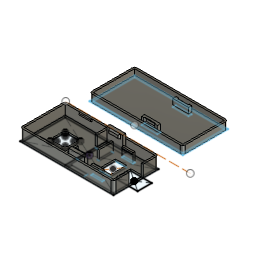
co2_01space_box (Autodesk Fusion 360 design; units mm, degrees)
Autodesk Fusion 360 part; units mm, degrees
sketch "Sketch7" plane through (0, 0, 0) normal (0, 0, 1) x (1, 0, 0)
  line L0 (28.4, 13.1) -> (-28.4, 13.1)
  line L1 (-28.4, 13.1) -> (-28.4, -13.1)
  line L2 (-28.4, -13.1) -> (28.4, -13.1)
  line L3 (28.4, -13.1) -> (28.4, 13.1)
  line L4 (28.4, 13.1) -> (-28.4, -13.1) construction
  line L5 (-28.4, 13.1) -> (28.4, -13.1) construction
  line L6 (-29.6, -14.3) -> (29.6, -14.3)
  line L7 (29.6, -14.3) -> (29.6, 14.3)
  line L8 (29.6, 14.3) -> (-29.6, 14.3)
  line L9 (-29.6, 14.3) -> (-29.6, -14.3)
  line L10 (-28.4, 13.1) -> (-2.2, 13.1)
  line L11 (-2.2, 13.1) -> (-2.2, -13.1)
  line L12 (-2.2, -13.1) -> (-28.4, -13.1)
  line L13 (-28.4, -13.1) -> (-28.4, 13.1)
  line L14 (-18.1, 4.8) -> (-12.5, 4.8)
  line L15 (-10.5, 2.8) -> (-10.5, -2.8)
  line L16 (-12.5, -4.8) -> (-18.1, -4.8)
  line L17 (-20.1, -2.8) -> (-20.1, 2.8)
  arc A0 (-18.1, 4.8) -> (-20.1, 2.8) centre (-18.1, 2.8) ccw
  arc A1 (-10.5, 2.8) -> (-12.5, 4.8) centre (-12.5, 2.8) ccw
  arc A2 (-20.1, -2.8) -> (-18.1, -4.8) centre (-18.1, -2.8) ccw
  arc A3 (-12.5, -4.8) -> (-10.5, -2.8) centre (-12.5, -2.8) ccw
  line L18 (-2.2, 13.1) -> (-1, 13.1)
  line L19 (-1, 13.1) -> (-1, -13.1)
  line L20 (-1, -13.1) -> (-2.2, -13.1)
  line L21 (-2.2, -13.1) -> (-2.2, 13.1)
  line L22 (-2.2, 5.9651) -> (-1, 5.9651)
  line L23 (-1, 5.9651) -> (-1, -6)
  line L24 (-1, -6) -> (-2.2, -6)
  line L25 (-2.2, -6) -> (-2.2, 5.9651)
  line L26 (35.1, -4.5) -> (21.7, -4.5)
  line L27 (21.7, -4.5) -> (21.7, 4.5)
  line L28 (21.7, 4.5) -> (35.1, 4.5)
  line L29 (35.1, 4.5) -> (35.1, -4.5)
  line L30 (35.1, -4.5) -> (21.7, 4.5) construction
  line L31 (21.7, -4.5) -> (35.1, 4.5) construction
  line L32 (18.5, -5) -> (11.5, -5)
  line L33 (11.5, -5) -> (11.5, 5)
  line L34 (11.5, 5) -> (18.5, 5)
  line L35 (18.5, 5) -> (18.5, -5)
  line L36 (18.5, -5) -> (11.5, 5) construction
  line L37 (11.5, -5) -> (18.5, 5) construction
  line L38 (11.5, 10.4) -> (18.5, 10.4)
  line L39 (18.5, 10.4) -> (18.5, 9.2)
  line L40 (18.5, 9.2) -> (11.5, 9.2)
  line L41 (11.5, 9.2) -> (11.5, 10.4)
  line L42 (11.5, -9.2) -> (18.5, -9.2)
  line L43 (18.5, -9.2) -> (18.5, -10.4)
  line L44 (18.5, -10.4) -> (11.5, -10.4)
  line L45 (11.5, -10.4) -> (11.5, -9.2)
  line L46 (6.2, 0) -> (5, 0)
  line L47 (5, 0) -> (5, 9)
  line L48 (5, 9) -> (6.2, 9)
  line L49 (6.2, 9) -> (6.2, 0)
  line L50 (-37, 22) -> (42, 22) construction
  line L51 (0, 13.1) -> (10, 13.1)
  line L52 (10, 13.1) -> (10, 11.1)
  line L53 (10, 11.1) -> (0, 11.1)
  line L54 (0, 11.1) -> (0, 13.1)
  line L55 (0, -13.1) -> (10, -13.1)
  line L56 (10, -13.1) -> (10, -11.1)
  line L57 (10, -11.1) -> (0, -11.1)
  line L58 (0, -11.1) -> (0, -13.1)
  line L59 (-29.6, 29.7) -> (-29.6, 58.3)
  line L60 (29.6, 29.7) -> (-29.6, 29.7)
  line L61 (-28.4, 30.9) -> (-2.2, 30.9)
  line L62 (-28.4, 30.9) -> (-28.4, 57.1)
  line L63 (-28.4, 57.1) -> (28.4, 57.1)
  line L64 (-29.6, 58.3) -> (29.6, 58.3)
  line L65 (29.6, 58.3) -> (29.6, 29.7)
  line L66 (28.4, 57.1) -> (28.4, 30.9)
  line L67 (28.4, 30.9) -> (-28.4, 30.9)
  line L68 (0, 33.1) -> (10, 33.1)
  line L69 (10, 33.1) -> (10, 35.1)
  line L70 (10, 35.1) -> (0, 35.1)
  line L71 (0, 35.1) -> (0, 33.1)
  line L72 (0, 54.9) -> (10, 54.9)
  line L73 (10, 54.9) -> (10, 52.9)
  line L74 (10, 52.9) -> (0, 52.9)
  line L75 (0, 52.9) -> (0, 54.9)
  point P0 (-20.1, 4.8)
  point P1 (-10.5, 4.8)
  point P2 (-20.1, -4.8)
  point P3 (28.4, 0)
  point P4 (15, 0)
  dimension "d75" = 56.8
  dimension "d76" = 26.2
  dimension "d77" = 1.2
  dimension "d78" = 26.2
  dimension "d79" = 26.2
  dimension "d80" = 9.6
  dimension "d81" = 9.6
  dimension "d82" = 8.3
  dimension "d83" = 8.3
  dimension "d84" = 2
  dimension "d85" = 2
  dimension "d86" = 2
  dimension "d87" = 2
  dimension "d88" = 1.2
  dimension "d89" = 26.2
  dimension "d90" = 1.2
  dimension "d91" = 11.9651
  dimension "d92" = 13.4
  dimension "d93" = 9
  dimension "d94" = 7
  dimension "d95" = 10
  dimension "d96" = 6.7
  dimension "d101" = 7
  dimension "d102" = 1.2
  dimension "d103" = 4.2
  dimension "d104" = 7
  dimension "d105" = 1.2
  dimension "d106" = 4.2
  dimension "d107" = 1.2
  dimension "d108" = 9
  dimension "d109" = 5.3
  dimension "d131" = 10
  dimension "d132" = 2
  dimension "d133" = 2
  dimension "d134" = 2
  dimension "d135" = 10
  dimension "d136" = 2
  dimension "d143" = 2.2
  dimension "d144" = 2.2
  constraint horizontal L0
  constraint perpendicular L0 L1
  constraint parallel L0 L2
  constraint parallel L1 L3
  constraint coincident L4 origin
  constraint coincident L5 origin
  constraint horizontal L10
  constraint vertical L11
  constraint horizontal L12
  constraint vertical L13
  constraint horizontal L14
  constraint vertical L15
  constraint horizontal L16
  constraint vertical L17
  constraint coincident P0 L17
  constraint coincident P0 L14
  constraint tangent L17 A0
  constraint tangent L14 A0
  constraint coincident P1 L14
  constraint coincident P1 L15
  constraint tangent L14 A1
  constraint tangent L15 A1
  constraint coincident P2 L17
  constraint coincident P2 L16
  constraint tangent L17 A2
  constraint tangent L16 A2
  constraint tangent L16 A3
  constraint tangent L15 A3
  constraint horizontal L18
  constraint vertical L19
  constraint horizontal L20
  constraint vertical L21
  constraint horizontal L22
  constraint vertical L23
  constraint horizontal L24
  constraint vertical L25
  constraint coincident L11 L22.start
  constraint horizontal L26
  constraint perpendicular L26 L27
  constraint parallel L26 L28
  constraint parallel L27 L29
  constraint coincident L30 P3
  constraint coincident L31 P3
  constraint midpoint L3 P3
  constraint horizontal L32
  constraint perpendicular L32 L33
  constraint parallel L32 L34
  constraint parallel L33 L35
  constraint coincident L36 P4
  constraint coincident L37 P4
  constraint horizontal L38
  constraint vertical L39
  constraint horizontal L40
  constraint vertical L41
  constraint horizontal L42
  constraint vertical L43
  constraint horizontal L44
  constraint vertical L45
  constraint horizontal L46
  constraint vertical L47
  constraint horizontal L48
  constraint vertical L49
  constraint parallel L8 L50
  constraint horizontal L51
  constraint vertical L52
  constraint horizontal L53
  constraint vertical L54
  constraint midpoint L0 L51.start
  constraint horizontal L55
  constraint vertical L56
  constraint horizontal L57
  constraint vertical L58
  constraint midpoint L2 L55.start
  constraint symmetric L0.start L50 L66.end
  constraint symmetric L0.end L50 L61.start
  constraint symmetric L1.end L50 L62.end
  constraint symmetric L2.end L50 L63.end
  constraint symmetric L6.start L50 L59.end
  constraint symmetric L6.end L50 L64.end
  constraint symmetric L7.end L50 L60.start
  constraint symmetric L8.end L50 L59.start
  constraint symmetric L10.end L50 L61.end
  constraint horizontal L68
  constraint vertical L69
  constraint horizontal L70
  constraint vertical L71
  constraint horizontal L72
  constraint vertical L73
  constraint horizontal L74
  constraint vertical L75
  measures "d75" distance of L1.end L2.end
  measures "d76" distance of L0.end L1.end
  measures "d78" distance of L0.end L10.end
  measures "d79" distance of L0.end L1.end
  measures "d80" distance of P0 P1
  measures "d81" distance of P0 P2
  measures "d82" distance of L0 L14
  measures "d83" distance of L13 L17
  measures "d84" radius of A0
  measures "d85" radius of A1
  measures "d86" radius of A2
  measures "d87" radius of A3
  measures "d88" distance of L10.end L18.end
  measures "d89" distance of L10.end L11.end
  measures "d90" distance of L22.start L22.end
  measures "d91" distance of L22.start L24.end
  measures "d92" distance of L27.end L28.end
  measures "d93" distance of L26.end L27.end
  measures "d94" distance of L33.end L34.end
  measures "d95" distance of L32.end L33.end
  measures "d96" distance of L27 P4
  measures "d101" distance of L38.start L38.end
  measures "d102" distance of L38.start L40.end
  measures "d103" distance of L34 L40
  measures "d104" distance of L42.start L42.end
  measures "d105" distance of L42.start L44.end
  measures "d106" distance of L32 L42
  measures "d107" distance of L46.start L46.end
  measures "d108" distance of L46.start L48.end
  measures "d109" distance of L33 L49
  measures "d131" distance of L51.start L51.end
  measures "d132" distance of L51.start L53.end
  measures "d133" distance of L55.start L57.end
  measures "d134" distance of L68.start L70.end
  measures "d135" distance of L72.start L72.end
  measures "d136" distance of L72.start L74.end
  measures "d143" distance of L67 L68
  measures "d144" distance of L63 L72
extrude "Extrude26" add sketch "Sketch7" along normal blind 10.4 contours L0 L51 L52 L53 L54 | L2 L55 L56 L57 L58 makes body 1 at (6.6667, 11.1, 3.4667) makes body 2 at (3.3333, -13.1, 6.9333)
extrude "Extrude19" add sketch "Sketch7" along normal blind 6 separate body contours L38 L39 L40 L41 | L42 L43 L44 L45 | L46 L47 L48 L49 makes body 3 at (13.8333, 10.4, 2) makes body 4 at (5, 3, 2) makes body 5 at (16.1667, -10.4, 2)
extrude "Extrude18" add sketch "Sketch7" along normal blind 7.6 separate body contours L0 L1 L2 L3 L6 L7 L8 L9 L10 L12 L13 L18 L20 L26 L28 L51 L55 | L0 L11 L18 L19 L21 L22 | L2 L11 L19 L20 L21 L24 makes body 6
extrude "Extrude17" add sketch "Sketch7" along normal blind 1.2 separate body contours L0 L2 L3 L19 L23 L26 L27 L28 L52 L53 L54 L56 L57 L58 | L0 L51 L52 L53 L54 | L0 L1 L2 L10 L11 L12 L13 L21 L25 | L11 L19 L21 L22 L23 L24 L25 | L2 L55 L56 L57 L58 | L38 L39 L40 L41 | L42 L43 L44 L45 | L46 L47 L48 L49 makes body 7
sketch "Sketch8" plane through (0, 9.2, 0) normal (0, -1, 0) x (1, 0, 0)
  line L0 (11.5, 0) -> (18.5, 0)
  line L1 (18.5, 0) -> (18.5, 6)
  line L2 (18.5, 6) -> (11.5, 6)
  line L3 (11.5, 6) -> (11.5, 0)
  line L4 (11.5, 6) -> (18.5, 6)
  line L5 (18.5, 6) -> (18.5, 4.8)
  line L6 (18.5, 4.8) -> (11.5, 4.8)
  line L7 (11.5, 4.8) -> (11.5, 6)
  dimension "d112" = 1.2
  constraint horizontal L4
  constraint vertical L5
  constraint horizontal L6
  constraint vertical L7
  constraint coincident L2.end L3.start
  measures "d112" distance of L2.end L6.end
extrude "Extrude20" add sketch "Sketch8" along normal blind 0.6 draft -30 contours L1 L2 L3 L4 L5 L6 L7 bodies 3
sketch "Sketch9" plane through (0, -9.2, 0) normal (0, 1, 0) x (-1, 0, 0)
  line L0 (-18.5, 0) -> (-11.5, 0)
  line L1 (-11.5, 0) -> (-11.5, 6)
  line L2 (-11.5, 6) -> (-18.5, 6)
  line L3 (-18.5, 6) -> (-18.5, 0)
  line L4 (-18.5, 6) -> (-11.5, 6)
  line L5 (-11.5, 6) -> (-11.5, 4.8)
  line L6 (-11.5, 4.8) -> (-18.5, 4.8)
  line L7 (-18.5, 4.8) -> (-18.5, 6)
  dimension "d115" = 7
  dimension "d116" = 1.2
  constraint horizontal L4
  constraint vertical L5
  constraint horizontal L6
  constraint vertical L7
  constraint coincident L2.end L3.start
  measures "d115" distance of L2.end L1.end
  measures "d116" distance of L2.end L6.end
extrude "Extrude21" add sketch "Sketch9" along normal blind 0.6 draft -30 contours L1 L2 L3 L4 L5 L6 L7 bodies 5
sketch "Sketch10" plane through (0, -13.1, 0) normal (0, 1, 0) x (-1, 0, 0)
  line L0 (2.2, 0) -> (28.4, 0)
  line L1 (28.4, 0) -> (28.4, 7.6)
  line L2 (28.4, 7.6) -> (2.2, 7.6)
  line L3 (2.2, 7.6) -> (2.2, 0)
  line L4 (11.4015, 7.6) -> (19.4015, 7.6)
  line L5 (19.4015, 7.6) -> (19.4015, 6)
  line L6 (19.4015, 6) -> (11.4015, 6)
  line L7 (11.4015, 6) -> (11.4015, 7.6)
  dimension "d119" = 8
  dimension "d120" = 1.6
  constraint horizontal L4
  constraint vertical L5
  constraint horizontal L6
  constraint vertical L7
  constraint coincident L2 L4.start
  measures "d119" distance of L4.start L4.end
  measures "d120" distance of L4.start L6.end
extrude "Extrude22" add sketch "Sketch10" along normal blind 0.6 draft -30 contours L2 L4 L5 L6 L7 bodies 6
sketch "Sketch11" plane through (0, 13.1, 0) normal (0, -1, 0) x (1, 0, 0)
  line L0 (-28.4, 0) -> (-2.2, 0)
  line L1 (-2.2, 0) -> (-2.2, 7.6)
  line L2 (-2.2, 7.6) -> (-28.4, 7.6)
  line L3 (-28.4, 7.6) -> (-28.4, 0)
  line L4 (-19.374, 7.6) -> (-11.374, 7.6)
  line L5 (-11.374, 7.6) -> (-11.374, 6)
  line L6 (-11.374, 6) -> (-19.374, 6)
  line L7 (-19.374, 6) -> (-19.374, 7.6)
  dimension "d123" = 8
  dimension "d124" = 1.6
  constraint horizontal L4
  constraint vertical L5
  constraint horizontal L6
  constraint vertical L7
  constraint coincident L2 L4.start
  measures "d123" distance of L4.start L4.end
  measures "d124" distance of L4.start L6.end
extrude "Extrude23" add sketch "Sketch11" along normal blind 0.6 draft -30 contours L2 L4 L5 L6 L7 bodies 6
fillet "Fillet7" radius 1.6 2 edges at (-29.6, 14.3, 3.8) (-29.6, -14.3, 3.8) on bodies 6
fillet "Fillet8" radius 1.6 2 edges at (29.6, -14.3, 3.8) (29.6, 14.3, 3.8) on bodies 6
extrude "Extrude24" add sketch "Sketch7" along normal blind 1.2 separate body contours L61 L62 L63 L66 L67 makes body 8
extrude "Extrude25" add sketch "Sketch7" along normal blind 4.8 contours L59 L60 L64 L65 | L68 L69 L70 L71 | L72 L73 L74 L75 bodies 8
sketch "Sketch12" plane through (0, 33.1, 0) normal (0, -1, 0) x (1, 0, 0)
  line L0 (0, 1.2) -> (10, 1.2)
  line L1 (10, 1.2) -> (10, 4.8)
  line L2 (10, 4.8) -> (0, 4.8)
  line L3 (0, 4.8) -> (0, 1.2)
  line L4 (1.3752, 4.8) -> (8.3752, 4.8)
  line L5 (8.3752, 4.8) -> (8.3752, 2)
  line L6 (8.3752, 2) -> (1.3752, 2)
  line L7 (1.3752, 2) -> (1.3752, 4.8)
  dimension "d145" = 7
  dimension "d146" = 2.8
  constraint horizontal L4
  constraint vertical L5
  constraint horizontal L6
  constraint vertical L7
  constraint coincident L2 L4.start
  measures "d145" distance of L4.start L4.end
  measures "d146" distance of L4.start L6.end
sketch "Sketch13" plane through (0, 54.9, 0) normal (0, 1, 0) x (-1, 0, 0)
  line L0 (-10, 1.2) -> (0, 1.2)
  line L1 (0, 1.2) -> (0, 4.8)
  line L2 (0, 4.8) -> (-10, 4.8)
  line L3 (-10, 4.8) -> (-10, 1.2)
  line L4 (-8.5822, 4.8) -> (-1.5822, 4.8)
  line L5 (-1.5822, 4.8) -> (-1.5822, 2)
  line L6 (-1.5822, 2) -> (-8.5822, 2)
  line L7 (-8.5822, 2) -> (-8.5822, 4.8)
  dimension "d149" = 7
  dimension "d150" = 2.8
  constraint horizontal L4
  constraint vertical L5
  constraint horizontal L6
  constraint vertical L7
  constraint coincident L2 L4.start
  measures "d149" distance of L4.start L4.end
  measures "d150" distance of L4.start L6.end
extrude "Extrude27" cut sketch "Sketch12" against normal blind 1 draft -30 contours L2 L4 L5 L6 L7 bodies 8
extrude "Extrude28" cut sketch "Sketch13" against normal blind 1 draft -30 contours L2 L4 L5 L6 L7 bodies 8
sketch "Sketch14" plane through (0, 11.1, 0) normal (0, -1, 0) x (1, 0, 0)
  line L0 (0, 0) -> (10, 0)
  line L1 (10, 0) -> (10, 10.4)
  line L2 (10, 10.4) -> (0, 10.4)
  line L3 (0, 10.4) -> (0, 0)
  line L4 (1.6418, 10.4) -> (8.6418, 10.4)
  line L5 (8.6418, 10.4) -> (8.6418, 7.6)
  line L6 (8.6418, 7.6) -> (1.6418, 7.6)
  line L7 (1.6418, 7.6) -> (1.6418, 10.4)
  dimension "d153" = 7
  dimension "d154" = 2.8
  constraint horizontal L4
  constraint vertical L5
  constraint horizontal L6
  constraint vertical L7
  constraint coincident L2 L4.start
  measures "d153" distance of L4.start L4.end
  measures "d154" distance of L4.start L6.end
extrude "Extrude29" add sketch "Sketch14" along normal blind 1 draft -30 contours L2 L4 L5 L6 L7 bodies 1
sketch "Sketch15" plane through (0, -11.1, 0) normal (0, 1, 0) x (-1, 0, 0)
  line L0 (-10, 0) -> (0, 0)
  line L1 (0, 0) -> (0, 10.4)
  line L2 (0, 10.4) -> (-10, 10.4)
  line L3 (-10, 10.4) -> (-10, 0)
  line L4 (-8.5743, 10.4) -> (-1.5743, 10.4)
  line L5 (-1.5743, 10.4) -> (-1.5743, 7.6)
  line L6 (-1.5743, 7.6) -> (-8.5743, 7.6)
  line L7 (-8.5743, 7.6) -> (-8.5743, 10.4)
  dimension "d157" = 7
  dimension "d158" = 2.8
  constraint horizontal L4
  constraint vertical L5
  constraint horizontal L6
  constraint vertical L7
  constraint coincident L2 L4.start
  measures "d157" distance of L4.start L4.end
  measures "d158" distance of L4.start L6.end
extrude "Extrude30" add sketch "Sketch15" along normal blind 1 draft -30 contours L2 L4 L5 L6 L7 bodies 2
chamfer "Chamfer1" distance 0.6 angle 45 1 edges at (5.0822, 54.9, 4.8) on bodies 8
chamfer "Chamfer2" distance 0.6 angle 45 1 edges at (4.8752, 33.1, 4.8) on bodies 8
fillet "Fillet9" radius 1.6 2 edges at (-29.6, 58.3, 2.4) (-29.6, 29.7, 2.4) on bodies 8
fillet "Fillet10" radius 1.6 2 edges at (29.6, 29.7, 2.4) (29.6, 58.3, 2.4) on bodies 8
